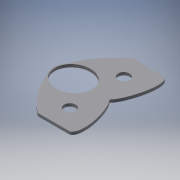
# Autodesk Inventor part: mocowanie_podwozia_gora
Saved by Autodesk Inventor 2017 (Build 210142000, 142)
## iProperties
Created: 2017-05-12
Part Number: mocowanie_podwozia_gora
Material: Ogólny
Document SubType Name: Modeling
Designer: Kuba01
Density: 1 g/cm^3
Appearance: Domyślna
Author: Kuba01
Autodesk Inventor part; units mm, degrees
ref_plane "YZ Plane" through (0, 0, 0) normal (1, 0, 0) x (0, 1, 0)
ref_plane "XZ Plane" through (0, 0, 0) normal (0, 1, 0) x (-1, 0, 0)
ref_plane "XY Plane" through (0, 0, 0) normal (0, 0, 1) x (1, 0, 0)
sketch "Szkic1" plane through (0, 0, 0) normal (0, 0, 1) x (1, 0, 0)
  circle A0 centre (0.2713, 9.4144) radius 2 projected
  circle A1 centre (0.2713, -9.4144) radius 2 projected
  ellipse E0 centre (-8.3642, 0) end of major axis (-1.8423, 0) minor radius 6 (-14.886, 0) -> (-13.7374, -3.4005) ccw projected
  spline S0 degree 3 poles (-3.8083, -16.5118) (-7.4967, -13.768) (-11.3809, -9.2364) (-13.7374, -3.4005) knots 1 1 1 1 1.842723 1.842723 1.842723 1.842723 projected
  line L0 (7.3687, -16.5118) -> (-3.8083, -16.5118) projected
  spline S1 degree 3 poles (4.6424, 0) (7.5886, -2.9462) (10.6572, -15.0638) (7.3687, -16.5118) knots 1 1 1 1 2 2 2 2 projected
  spline S2 degree 3 poles (7.3687, 16.5118) (10.6572, 15.0638) (7.5886, 2.9462) (4.6424, 0) knots 1 1 1 1 2 2 2 2 projected
  line L1 (-3.8083, 16.5118) -> (7.3687, 16.5118) projected
  spline S3 degree 3 poles (-13.7374, 3.4005) (-11.3809, 9.2364) (-7.4967, 13.768) (-3.8083, 16.5118) knots 1.157277 1.157277 1.157277 1.157277 2 2 2 2 projected
  ellipse E1 centre (-8.3642, 0) end of major axis (-1.8423, 0) minor radius 6 (-13.7374, 3.4005) -> (-14.886, 0) ccw projected
  ellipse E2 centre (-7.9381, 0) end of major axis (-1.4162, 0) minor radius 6 projected
  point P0 (0, 0)
  constraints: 3 other
extrude "Wyciągnięcie proste1" add sketch "Szkic1" along normal blind 1
